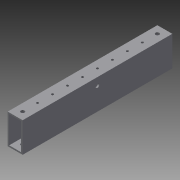
# Autodesk Inventor part: frame_side_bumper
Saved by Autodesk Inventor 2015 SP1 (Build 190203100, 203)
## iProperties
Created: 2014-12-23
Part Number: frame_side_bumper
Material: Generic
Document SubType Name: Modeling
Designer: Jarod
Density: 1 g/cm^3
Appearance: Default
Author: Jarod
Autodesk Inventor part; units mm, degrees
ref_plane "YZ Plane" through (0, 0, 0) normal (1, 0, 0) x (0, 1, 0)
ref_plane "XZ Plane" through (0, 0, 0) normal (0, 1, 0) x (-1, 0, 0)
ref_plane "XY Plane" through (0, 0, 0) normal (0, 0, 1) x (1, 0, 0)
sketch "Sketch1" plane through (0, 0, 0) normal (0, 0, 1) x (1, 0, 0)
  line L0 (0, 0) -> (25.4, 0)
  line L1 (25.4, 0) -> (25.4, 50.8)
  line L2 (25.4, 50.8) -> (0, 50.8)
  line L3 (0, 50.8) -> (0, 0)
  line L4 (2.54, 2.54) -> (22.86, 2.54)
  line L5 (22.86, 2.54) -> (22.86, 48.26)
  line L6 (22.86, 48.26) -> (2.54, 48.26)
  line L7 (2.54, 48.26) -> (2.54, 2.54)
  dimension "d0" = 25.4
  dimension "d1" = 50.8
  dimension "d2" = 20.32
  dimension "d3" = 45.72
  dimension "d4" = 2.54
  dimension "d5" = 2.54
  constraints: 16 end point, 4 parallel, 2 horizontal, 2 perpendicular
  measures "d0" distance of L2.end L1.end
  measures "d1" distance of L1.end L0.end
  measures "d2" distance of L6.end L5.end
  measures "d3" distance of L5.end L4.end
  measures "d4" distance between parallel lines of L0 L4
  measures "d5" distance between parallel lines of L3 L7
extrude "Extrusion1" add sketch "Sketch1" along normal blind 254
sketch "Sketch2" plane through (0, 50.8, 0) normal (0, 1, 0) x (1, 0, 0)
  line L0 (25.4, 0) -> (0, 0) projected
  line L1 (0, 0) -> (0, -254) projected
  line L2 (25.4, -254) -> (0, -254) projected
  line L3 (25.4, 0) -> (25.4, -254) projected
  point P0 (12.7, -12.7)
  dimension "d8" = 12.7
  dimension "d9" = 12.7
  measures "d8" distance from line of L1 point (12.7, -12.7)
  measures "d9" distance from line of L0 point (12.7, -12.7)
hole "Hole1" at (12.7, 50.8, 12.7) direction (0, -1, 0) diameter 3.9688 end through all
pattern_linear "Rectangular Pattern1" count 10 spacing 25.4 along (0, 0, 1) of "Hole1"
sketch "Sketch3" plane through (0, 50.8, 0) normal (0, 1, 0) x (1, 0, 0)
  circle A0 centre (12.7, -241.3) radius 1.9844 projected
  circle A1 centre (12.7, -215.9) radius 1.9844 projected
  circle A2 centre (12.7, -190.5) radius 1.9844 projected
  circle A3 centre (12.7, -165.1) radius 1.9844 projected
  circle A4 centre (12.7, -139.7) radius 1.9844 projected
  circle A5 centre (12.7, -114.3) radius 1.9844 projected
  circle A6 centre (12.7, -88.9) radius 1.9844 projected
  circle A7 centre (12.7, -63.5) radius 1.9844 projected
  circle A8 centre (12.7, -38.1) radius 1.9844 projected
  circle A9 centre (12.7, -12.7) radius 1.9844 projected
  line L0 (25.4, 0) -> (0, 0) projected
  line L1 (0, 0) -> (0, -254) projected
  line L2 (25.4, -254) -> (0, -254) projected
  line L3 (25.4, 0) -> (25.4, -254) projected
  circle A10 centre (12.7, -12.7) radius 3.175
  circle A11 centre (12.7, -241.3) radius 3.175
  dimension "d20" = 6.35
  dimension "d21" = 6.35
  constraints: 2 centre point, 2 coincident
  measures "d20" diameter of A10
  measures "d21" diameter of A11
extrude "Extrusion2" cut sketch "Sketch3" against normal blind 279.4 contours A0 | A9 | A10 | A11
sketch "Sketch4" plane through (25.4, 0, 0) normal (1, 0, 0) x (0, 0, -1)
  line L0 (0, 0) -> (0, 50.8) projected
  line L1 (0, 50.8) -> (-254, 50.8) projected
  line L2 (-254, 0) -> (-254, 50.8) projected
  line L3 (0, 0) -> (-254, 0) projected
  point P0 (-127, 38.1)
  dimension "d24" = 12.7
  dimension "d25" = 127
  measures "d24" distance from line of L1 point (-127, 38.1)
  measures "d25" distance from line of point (-127, 38.1) L2
hole "Hole2" at (25.4, 38.1, 127) direction (-1, 0, 0) diameter 6.35 end through all
body "Solid1"
